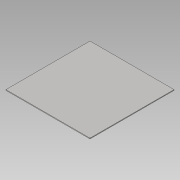
# Autodesk Inventor part: Ceiling
Saved by Autodesk Inventor 2016 (Build 200138000, 138)
## iProperties
Created: 2017-05-19
Part Number: Ceiling
Material: Generic
Document SubType Name: Modeling
Designer: 31745
Density: 1 g/cm^3
Appearance: Default
Author: 31745
Autodesk Inventor part; units mm, degrees
ref_plane "YZ Plane" through (0, 0, 0) normal (1, 0, 0) x (0, 1, 0)
ref_plane "XZ Plane" through (0, 0, 0) normal (0, 1, 0) x (-1, 0, 0)
ref_plane "XY Plane" through (0, 0, 0) normal (0, 0, 1) x (1, 0, 0)
sketch "Sketch1" plane through (0, 0, 0) normal (0, 1, 0) x (-1, 0, 0)
  line L0 (0, 0) -> (-254, 0)
  line L1 (-254, 0) -> (-254, -254)
  line L2 (-254, -254) -> (0, -254)
  line L3 (0, -254) -> (0, 0)
  dimension "d0" = 254
  dimension "d1" = 254
  constraints: 8 end point, 2 parallel, 1 horizontal, 1 perpendicular
  measures "d0" distance of L2.end L1.end
  measures "d1" distance of L1.end L0.end
extrude "Extrusion1" add sketch "Sketch1" against normal blind 2.286
body "Solid1"
